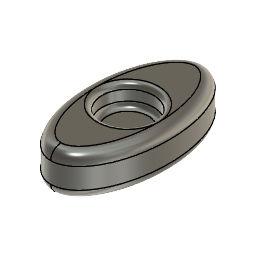
Nose-Pad (Autodesk Fusion 360 design; units mm, degrees)
part number: 2026-05-19-13-18-48-388
Autodesk Fusion 360 part; units mm, degrees
sketch "Sketch1" plane through (0, 0, 0) normal (0, 0, 1) x (1, 0, 0)
  ellipse E0 centre (0, 0) end of major axis (0, 7.5) minor radius 4
  line L0 (0, -7.5) -> (0, 7.5) construction
  line L1 (4, 0) -> (-4, 0) construction
  dimension "d1" = 15
  dimension "d2" = 8
  constraint coincident E0 L0.start
  constraint coincident E0 L0.end
  constraint coincident E0 L1.start
  constraint coincident E0 L1.end
  constraint coincident E0.centre origin
  constraint vertical L0
  measures "d1" distance of E0
extrude "Extrude1" add sketch "Sketch1" along normal blind 4
fillet "Fillet1" radius 1 1 faces at (-1.3236, 0.0107, 4)
fillet "Fillet2" radius 1 1 faces at (-1.3236, 0.0107, 0)
sketch "Sketch2" plane through (0, 0, 4) normal (0, 0, 1) x (-1, 0, 0)
  spline S0 degree 3 poles (0, 6.5) (0.1564, 6.5) (0.3119, 6.4662) (0.6708, 6.3245) (0.8631, 6.1929) (1.358, 5.7588) (1.6148, 5.4081) (2.2677, 4.2924) (2.5437, 3.4618) (2.8895, 1.8705) (2.9754, 1.1073) (3.0147, -0.3882) (2.9734, -1.1223) (2.7876, -2.3869) (2.6722, -2.9212) (2.3792, -3.8773) (2.2153, -4.3037) (1.8676, -4.9911) (1.7055, -5.2626) (1.3451, -5.7425) (1.1515, -5.9556) (0.7579, -6.2645) (0.5702, -6.3765) (0.2152, -6.4892) (0.0561, -6.5094) (-0.1918, -6.4875) (-0.2818, -6.4684) (-0.687, -6.3384) (-0.9609, -6.1288) (-1.5465, -5.5328) (-1.8165, -5.1021) (-2.4831, -3.7522) (-2.7377, -2.7673) (-3.0012, -0.8941) (-3.0304, -0.0028) (-2.9314, 1.4501) (-2.8553, 2.0161) (-2.6454, 3.0019) (-2.529, 3.4248) (-2.277, 4.1304) (-2.1564, 4.4188) (-1.8857, 4.9565) (-1.7386, 5.2073) (-1.4536, 5.6032) (-1.3274, 5.7567) (-1.0487, 6.0386) (-0.896, 6.1674) (-0.6081, 6.3456) (-0.4806, 6.407) (-0.2341, 6.4813) (-0.1172, 6.5) (0, 6.5) knots -3.141593 -3.141593 -3.141593 -3.141593 -3.045564 -3.045564 -2.90463 -2.90463 -2.641285 -2.641285 -2.110746 -2.110746 -1.641185 -1.641185 -1.191441 -1.191441 -0.856163 -0.856163 -0.5769 -0.5769 -0.3833 -0.3833 -0.208122 -0.208122 -0.076037 -0.076037 0.020583 0.020583 0.076788 0.076788 0.281874 0.281874 0.589921 0.589921 1.206479 1.206479 1.75165 1.75165 2.101341 2.101341 2.370334 2.370334 2.562138 2.562138 2.739908 2.739908 2.861709 2.861709 2.98347 2.98347 3.069636 3.069636 3.141593 3.141593 3.141593 3.141593
  circle A0 centre (0, 0) radius 2.5
  dimension "d9" = 5
  constraint coincident A0.centre origin
  measures "d9" diameter of A0
extrude "Extrude2" cut sketch "Sketch2" against normal blind 2 contours A0
fillet "Fillet5" radius 0.5 1 edges at (2.3308, -0.904, 4)
fillet "Fillet6" radius 0.5 1 edges at (2.3308, -0.904, 2)
